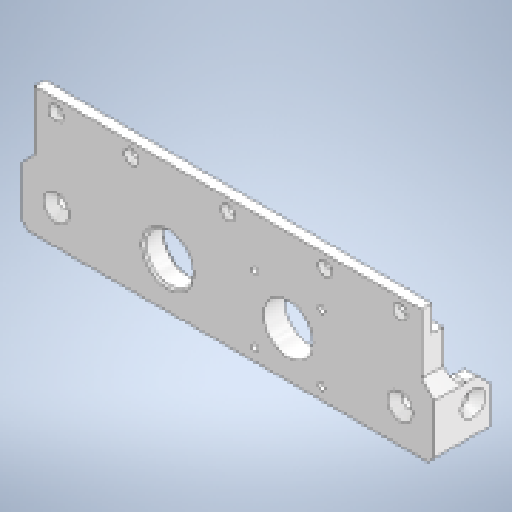
# Autodesk Inventor part: wall
Saved by Autodesk Inventor 2024 (Build 280153000, 153)
## iProperties
Created: 2023-08-11
Part Number: wall
Material: ABS Plastic
Document SubType Name: Modeling
Designer: l1534
Density: 1.06 g/cm^3
Appearance: Smooth - White
Author: l1534
Autodesk Inventor part; units mm, degrees
ref_plane "YZ Plane" through (0, 0, 0) normal (1, 0, 0) x (0, 1, 0)
ref_plane "XZ Plane" through (0, 0, 0) normal (0, 1, 0) x (-1, 0, 0)
ref_plane "XY Plane" through (0, 0, 0) normal (0, 0, 1) x (1, 0, 0)
sketch "Sketch1" plane through (0, 0, 0) normal (0, 0, 1) x (1, 0, 0)
  line L0 (-96.9802, 31.1578) -> (83.0198, 31.1578)
  line L1 (83.0198, 31.1578) -> (83.0198, -28.8422)
  line L2 (83.0198, -28.8422) -> (-96.9802, -28.8422)
  line L3 (-96.9802, -28.8422) -> (-96.9802, 31.1578)
  point P0 (0, 0)
  dimension "d0" = 180
  dimension "d1" = 60
  constraints: 8 end point, 2 parallel, 1 horizontal, 1 perpendicular
  measures "d0" distance of L0.start L0.end
  measures "d1" distance of L0.end L1.end
extrude "Extrusion1" add sketch "Sketch1" along normal blind 10
sketch "Sketch4" plane through (0, 0, 0) normal (0, 0, -1) x (-1, 0, 0)
  circle A0 centre (-21.0198, -7.6922) radius 11.5
  line L0 (96.9802, -28.8422) -> (-83.0198, -28.8422) projected
  line L1 (-83.0198, -28.8422) -> (-83.0198, 31.1578) projected
  point P0 (0, 0)
  dimension "d16" = 23
  dimension "d17" = 21.15
  dimension "d18" = 62
  constraints: 1 centre point
  measures "d16" diameter of A0
  measures "d17" distance from line of L0 A0.centre
  measures "d18" distance from line of L1 A0.centre
extrude "Extrusion4" cut sketch "Sketch4" against normal through all
sketch "Sketch5" plane through (0, 0, 0) normal (0, 0, -1) x (-1, 0, 0)
  line L0 (96.9802, -28.8422) -> (-83.0198, -28.8422) projected
  line L1 (96.9802, 31.1578) -> (96.9802, -28.8422) projected
  line L2 (-83.0198, -28.8422) -> (96.9802, -28.8422)
  line L3 (96.9802, -28.8422) -> (96.9802, -22.8422)
  line L4 (96.9802, -22.8422) -> (-83.0198, -22.8422)
  line L5 (-83.0198, -22.8422) -> (-83.0198, -28.8422)
  point P0 (0, 0)
  dimension "d21" = 6
  constraints: 8 end point, 2 parallel, 1 horizontal, 1 perpendicular, 1 point on line
  measures "d21" distance between parallel lines of L0 L4
extrude "Extrusion5" add sketch "Sketch5" along normal blind 16
sketch "Sketch6" plane through (-96.9802, -22.8422, 0) normal (0, 1, 0) x (1, 0, 0)
  line L0 (180, 16) -> (0, 16) projected
  line L1 (180, 0) -> (0, 0) projected
  line L2 (165.9, 16) -> (159.9, 16)
  line L3 (159.9, 16) -> (159.9, 0)
  line L4 (159.9, 0) -> (165.9, 0)
  line L5 (165.9, 0) -> (165.9, 16)
  line L6 (14.1, 16) -> (20.1, 16)
  line L7 (20.1, 16) -> (20.1, 0)
  line L8 (20.1, 0) -> (14.1, 0)
  line L9 (14.1, 0) -> (14.1, 16)
  line L10 (0, 0) -> (0, 16) projected
  line L11 (180, 0) -> (180, 16) projected
  point P0 (96.9802, 0)
  point P1 (14.1, 16)
  point P2 (14.1, 0)
  point P3 (20.1, 16)
  point P4 (165.9, 0)
  dimension "d24" = 14.1
  dimension "d25" = 6
  dimension "d26" = 14.1
  dimension "d27" = 6
  constraints: 16 end point, 4 parallel, 4 point on line, 2 horizontal, 2 perpendicular
  measures "d24" distance between parallel lines of L10 L9
  measures "d25" distance between parallel lines of L7 L9
  measures "d26" distance between parallel lines of L11 L5
  measures "d27" distance between parallel lines of L5 L3
extrude "Extrusion6" add sketch "Sketch6" along normal blind 20 contours L5 L1 L3 L0 | L7 L1 L9 L0
sketch "Sketch7" plane through (-76.8802, -22.8422, 0) normal (0, 1, 0) x (1, 0, 0)
  line L0 (0, 16) -> (139.8, 16) projected
  line L1 (0, 16) -> (0, 0) projected
  line L2 (139.8, 16) -> (0, 16)
  line L3 (0, 16) -> (0, 0)
  line L4 (0, 0) -> (139.8, 0)
  line L5 (139.8, 0) -> (139.8, 16)
  point P0 (76.8802, 0)
  constraints: 8 end point, 2 parallel, 1 horizontal, 1 perpendicular
extrude "Extrusion7" cut sketch "Sketch7" against normal through all
chamfer "Chamfer1" distance 3 angle 45 2 edges at (62.9198, -28.8422, -8) (-76.8802, -28.8422, -8)
sketch "Sketch8" plane through (0, 0, 10) normal (0, 0, 1) x (1, 0, 0)
  circle A0 centre (-34.9802, -7.6922) radius 11.05
  line L0 (-96.9802, -28.8422) -> (83.0198, -28.8422) projected
  line L1 (-96.9802, 31.1578) -> (-96.9802, -28.8422) projected
  point P0 (0, 0)
  dimension "d35" = 22.1
  dimension "d36" = 21.15
  dimension "d37" = 62
  constraints: 1 centre point
  measures "d35" diameter of A0
  measures "d36" distance from line of L0 A0.centre
  measures "d37" distance from line of L1 A0.centre
extrude "Extrusion8" cut sketch "Sketch8" against normal through all
chamfer "Chamfer2" distance 1 angle 45 2 edges at (-46.0302, -7.6922, 10) (-46.0302, -7.6922, 0)
sketch "Sketch9" plane through (-96.9802, -28.8422, 10) normal (0, -1, 0) x (1, 0, 0)
  circle A0 centre (10, -18) radius 2
  circle A1 centre (170, -18) radius 2
  line L0 (180, -26) -> (180, 0) projected
  line L1 (0, 0) -> (0, -26) projected
  line L2 (17.1, -26) -> (0, -26) projected
  line L3 (180, -26) -> (162.9, -26) projected
  point P0 (96.9802, -10)
  dimension "d43" = 4
  dimension "d44" = 10
  dimension "d45" = 4
  dimension "d46" = 10
  dimension "d47" = 8
  dimension "d48" = 8
  constraints: 2 centre point
  measures "d43" diameter of A1
  measures "d44" distance from line of L0 A1.centre
  measures "d45" diameter of A0
  measures "d46" distance from line of L1 A0.centre
  measures "d47" distance from line of L2 A0.centre
  measures "d48" distance from line of L3 A1.centre
extrude "Extrusion9" cut sketch "Sketch9" against normal through all
chamfer "Chamfer3" distance 3.5 angle 45 2 edges at (71.0198, -28.8422, -8) (-88.9802, -28.8422, -8)
sketch "Sketch10" plane through (0, 0, 10) normal (0, 0, 1) x (1, 0, 0)
  circle A0 centre (-86.9802, 25.1578) radius 1.5
  circle A1 centre (-51.9802, 25.1578) radius 1.5
  circle A2 centre (-6.9802, 25.1578) radius 1.5
  circle A3 centre (38.0198, 25.1578) radius 1.5
  circle A4 centre (73.0198, 25.1578) radius 1.5
  line L0 (83.0198, 31.1578) -> (-96.9802, 31.1578) projected
  line L1 (83.0198, -28.8422) -> (83.0198, 31.1578) projected
  line L2 (-96.9802, 31.1578) -> (-96.9802, -28.8422) projected
  point P0 (0, 0)
  dimension "d54" = 3
  dimension "d55" = 3
  dimension "d56" = 3
  dimension "d57" = 3
  dimension "d58" = 3
  dimension "d59" = 6
  dimension "d60" = 6
  dimension "d61" = 6
  dimension "d62" = 6
  dimension "d63" = 6
  dimension "d64" = 10
  dimension "d65" = 10
  dimension "d66" = 35
  dimension "d67" = 35
  dimension "d68" = 90
  constraints: 5 centre point
  measures "d54" diameter of A4
  measures "d55" diameter of A3
  measures "d56" diameter of A2
  measures "d57" diameter of A1
  measures "d58" diameter of A0
  measures "d59" distance from line of L0 A1.centre
  measures "d60" distance from line of L0 A0.centre
  measures "d61" distance from line of L0 A2.centre
  measures "d62" distance from line of L0 A3.centre
  measures "d63" distance from line of L0 A4.centre
  measures "d64" distance from line of L1 A4.centre
  measures "d65" distance from line of L2 A0.centre
  measures "d66" distance of A0.centre A1.centre
  measures "d67" distance of A4.centre A3.centre
  measures "d68" distance from line of L1 A2.centre
extrude "Extrusion10" cut sketch "Sketch10" against normal through all
chamfer "Chamfer4" distance 1.8 angle 45 5 edges at (-88.4802, 25.1578, 10) (-53.4802, 25.1578, 10) (-8.4802, 25.1578, 10) (36.5198, 25.1578, 10) (71.5198, 25.1578, 10)
sketch "Sketch11" plane through (-96.9802, -22.8422, -16) normal (-1, 0, 0) x (0, 0, 1)
  circle A0 centre (8, 10) radius 2
  line L0 (16, 0) -> (0, 0) projected
  line L1 (0, 0) -> (0, 20) projected
  point P0 (16, 22.8422)
  dimension "d77" = 4
  dimension "d78" = 10
  dimension "d79" = 8
  constraints: 1 centre point
  measures "d77" diameter of A0
  measures "d78" distance from line of L0 A0.centre
  measures "d79" distance from line of L1 A0.centre
extrude "Extrusion11" cut sketch "Sketch11" against normal through all
chamfer "Chamfer6" distance 3 angle 45 2 edges at (62.9198, -12.8422, -10) (-76.8802, -12.8422, -10)
sketch "Sketch12" plane through (0, 0, 0) normal (0, 0, -1) x (-1, 0, 0)
  circle A0 centre (-36.5198, 7.8078) radius 1.5
  circle A1 centre (-5.5198, 7.8078) radius 1.5
  circle A2 centre (-5.5198, -23.1922) radius 1.5
  circle A3 centre (-36.5198, -23.1922) radius 1.5
  circle A4 centre (-21.0198, -7.6922) radius 11.5 projected
  point P0 (0, 0)
  dimension "d85" = 3
  dimension "d86" = 3
  dimension "d87" = 3
  dimension "d88" = 3
  dimension "d89" = 15.5
  dimension "d90" = 15.5
  dimension "d91" = 15.5
  dimension "d93" = 15.5
  dimension "d94" = 15.5
  dimension "d95" = 15.5
  dimension "d96" = 31
  dimension "d97" = 15.5
  constraints: 4 centre point
  measures "d85" diameter of A0
  measures "d86" diameter of A1
  measures "d87" diameter of A3
  measures "d88" diameter of A2
  measures "d89" horizontal distance of A4.centre A1.centre
  measures "d90" horizontal distance of A0.centre A4.centre
  measures "d91" horizontal distance of A4.centre A3.centre
  measures "d93" horizontal distance of A4.centre A2.centre
  measures "d94" horizontal distance of A4.centre A1.centre
  measures "d95" horizontal distance of A4.centre A0.centre
  measures "d96" distance of A2.centre A3.centre
  measures "d97" horizontal distance of A4.centre A2.centre
extrude "Extrusion12" cut sketch "Sketch12" against normal through all contours A0 | A1 | A2 | A3
chamfer "Chamfer7" distance 1.8 angle 45 4 edges at (38.0198, 7.8078, 0) (7.0198, 7.8078, 0) (7.0198, -23.1922, 0) (38.0198, -23.1922, 0)
sketch "Sketch13" plane through (-96.9802, -22.8422, -16) normal (-1, 0, 0) x (0, 0, 1)
  line L0 (16, 0) -> (16, 54) projected
  line L1 (16, 41.9) -> (21.1, 41.9)
  line L2 (21.1, 41.9) -> (21.1, 54)
  line L3 (21.1, 54) -> (16, 54)
  line L4 (16, 54) -> (16, 41.9)
  line L5 (26, 54) -> (16, 54) projected
  point P0 (16, 22.8422)
  point P1 (16, 52)
  point P2 (16, 52)
  dimension "d103" = 12.1
  dimension "d104" = 12.1
  dimension "d105" = 5.1
  constraints: 8 end point, 2 parallel, 1 horizontal, 1 perpendicular, 1 point on line
  measures "d103" distance between parallel lines of L5 L1
  measures "d104" distance of L1.end L2.end
  measures "d105" distance of L2.end L0.end
extrude "Extrusion13" cut sketch "Sketch13" against normal through all
sketch "Sketch14" plane through (68.9198, -22.8422, 0) normal (1, 0, 0) x (0, 0, -1)
  line L0 (16, 20) -> (0, 20) projected
  line L1 (0, 0) -> (16, 0) projected
  line L2 (0, 20) -> (16, 20)
  line L3 (16, 20) -> (16, 0)
  line L4 (16, 0) -> (0, 0)
  line L5 (0, 0) -> (0, 20)
  point P0 (0, 22.8422)
  point P1 (16, 20)
  point P2 (0, 0)
  constraints: 8 end point, 2 parallel, 1 horizontal, 1 perpendicular
extrude "Extrusion14" cut sketch "Sketch14" against normal through all
sketch "Sketch15" plane through (83.0198, -28.8422, 10) normal (1, 0, 0) x (0, 0, -1)
  line L0 (0, 60) -> (0, 0) projected
  line L1 (0, 0) -> (26, 0)
  line L2 (26, 0) -> (26, 26.1)
  line L3 (26, 26.1) -> (0, 26.1)
  line L4 (0, 26.1) -> (0, 0)
  line L5 (10, 6) -> (26, 6) projected
  point P0 (10, 28.8422)
  point P1 (0, 26.1)
  dimension "d110" = 20.1
  dimension "d111" = 26
  constraints: 8 end point, 2 parallel, 1 horizontal, 1 perpendicular
  measures "d110" distance between parallel lines of L5 L3
  measures "d111" distance of L2.end L3.end
extrude "Extrusion15" add sketch "Sketch15" along normal blind 6
chamfer "Chamfer8" distance 6 angle 45 1 edges at (83.0198, -2.7422, 5)
chamfer "Chamfer9" distance 3 angle 45 1 edges at (89.0198, -28.8422, -3)
sketch "Sketch16" plane through (89.0198, -28.8422, 10) normal (1, 0, 0) x (0, 0, -1)
  circle A0 centre (18, 16.1) radius 2
  line L0 (26, 26.1) -> (10, 26.1) projected
  line L1 (26, 0) -> (26, 26.1) projected
  point P0 (10, 28.8422)
  point P1 (23, 26.1)
  dimension "d123" = 4
  dimension "d124" = 10
  dimension "d125" = 8
  constraints: 1 centre point
  measures "d123" diameter of A0
  measures "d124" distance from line of L0 A0.centre
  measures "d125" distance from line of L1 A0.centre
extrude "Extrusion16" cut sketch "Sketch16" against normal through all
chamfer "Chamfer11" distance 3.8 angle 45 1 edges at (89.0198, -12.7422, -6)
chamfer "Chamfer12" distance 6 angle 45 1 edges at (86.0198, -2.7422, -16)
sketch "Sketch17" plane through (-96.9802, -28.8422, 10) normal (-1, 0, 0) x (0, 0, 1)
  line L0 (0, 0) -> (-26, 0) projected
  line L1 (0, 0) -> (-26, 0)
  line L2 (-26, 0) -> (-26, 26.1)
  line L3 (-26, 26.1) -> (0, 26.1)
  line L4 (0, 26.1) -> (0, 0)
  point P0 (-10, 28.8422)
  dimension "d134" = 26
  dimension "d135" = 26.1
  constraints: 8 end point, 2 parallel, 1 horizontal, 1 perpendicular
  measures "d134" distance of L2.end L3.end
  measures "d135" distance of L1.end L2.end
extrude "Extrusion17" add sketch "Sketch17" along normal blind 6
chamfer "Chamfer13" distance 6 angle 45 1 edges at (-96.9802, -2.7422, 5)
chamfer "Chamfer14" distance 3 angle 45 1 edges at (-102.9802, -28.8422, -3)
chamfer "Chamfer15" distance 6 angle 45 1 edges at (-99.9802, -2.7422, -16)
sketch "Sketch18" plane through (-102.9802, -28.8422, 10) normal (-1, 0, 0) x (0, 0, 1)
  circle A0 centre (-18, 16.1) radius 2 projected
  circle A1 centre (-18, 16.1) radius 2
  point P0 (-10, 28.8422)
  constraints: 1 centre point, 1 coincident
extrude "Extrusion18" cut sketch "Sketch18" against normal through all
chamfer "Chamfer16" distance 3.5 angle 45 1 edges at (-102.9802, -12.7422, -10)
sketch "Sketch19" plane through (0, 0, 10) normal (0, 0, 1) x (1, 0, 0)
  circle A0 centre (-86.9802, -12.8422) radius 2.5
  circle A1 centre (73.0198, -12.8422) radius 2.5
  line L0 (-96.9802, 31.1578) -> (-96.9802, 3.2578) projected
  line L1 (86.0198, -28.8422) -> (-99.9802, -28.8422) projected
  line L2 (83.0198, 3.2578) -> (83.0198, 31.1578) projected
  point P0 (0, 0)
  dimension "d152" = 5
  dimension "d153" = 5
  dimension "d154" = 10
  dimension "d155" = 16
  dimension "d156" = 10
  dimension "d157" = 16
  constraints: 2 centre point
  measures "d152" diameter of A1
  measures "d153" diameter of A0
  measures "d154" distance from line of L0 A0.centre
  measures "d155" distance from line of L1 A0.centre
  measures "d156" distance from line of L2 A1.centre
  measures "d157" distance from line of L1 A1.centre
extrude "Extrusion19" cut sketch "Sketch19" against normal through all
chamfer "Chamfer17" distance 3.5 angle 45 2 edges at (-89.4802, -12.8422, 10) (70.5198, -12.8422, 10)
fillet "Fillet1" radius 5 2 edges at (-99.9802, -2.7422, 0) (86.0197, -2.7422, 0)
body "Solid1"
